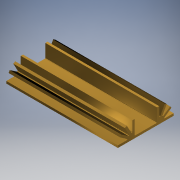
# Autodesk Inventor part: ZD3-5 Disipador
Saved by Autodesk Inventor 2018.3 (Build 223284000, 284)
## iProperties
Created: 2021-05-04
Part Number: ZD3-5 Disipador
Material: Latón, amarillo claro
Document SubType Name: Modeling
Designer: laguerre
Density: 8.47 g/cm^3
Appearance: Latón - Satinado
Author: laguerre
Autodesk Inventor part; units mm, degrees
ref_plane "YZ Plane" through (0, 0, 0) normal (1, 0, 0) x (0, 1, 0)
ref_plane "XZ Plane" through (0, 0, 0) normal (0, 1, 0) x (-1, 0, 0)
ref_plane "XY Plane" through (0, 0, 0) normal (0, 0, 1) x (1, 0, 0)
sketch "Boceto39" plane through (0, 0, 0) normal (0, 0, 1) x (1, 0, 0)
  line L0 (-25, 0) -> (25, 0)
  line L1 (10, 15) -> (10, 2.5)
  line L2 (9.5, 2) -> (-9.5, 2)
  line L3 (10, 15) -> (12, 15)
  line L4 (12, 15) -> (12, 6)
  line L5 (12.9398, 5.7622) -> (16.9826, 13.2392)
  line L6 (16.9826, 13.2392) -> (18.7419, 12.288)
  line L7 (18.7419, 12.288) -> (14.947, 5.2693)
  line L8 (15.67, 4.6194) -> (21.8509, 8.8675)
  line L9 (21.8509, 8.8675) -> (22.9837, 7.2192)
  line L10 (22.9837, 7.2192) -> (16.7168, 2.9121)
  line L11 (17, 2) -> (25, 2)
  line L12 (25, 2) -> (25, 0)
  line L13 (-10, 2.5) -> (-10, 14)
  line L14 (-10, 14) -> (-12, 14)
  line L15 (-17, 2) -> (-25, 2)
  line L16 (-25, 2) -> (-25, 0)
  arc A0 (25, 0) -> (10, 15) centre (10, 0) ccw construction
  line L17 (-12, 14) -> (-12, 6)
  line L18 (-12.9398, 5.7622) -> (-16.9826, 13.2392)
  line L19 (-16.9826, 13.2392) -> (-18.7419, 12.288)
  line L20 (-18.7419, 12.288) -> (-14.947, 5.2693)
  line L21 (-15.67, 4.6194) -> (-21.8509, 8.8675)
  line L22 (-21.8509, 8.8675) -> (-22.9837, 7.2192)
  line L23 (-22.9837, 7.2192) -> (-16.7168, 2.9121)
  arc A1 (-12.9398, 5.7622) -> (-12, 6) centre (-12.5, 6) ccw
  arc A2 (-15.67, 4.6194) -> (-14.947, 5.2693) centre (-15.3868, 5.0315) ccw
  arc A3 (-17, 2) -> (-16.7168, 2.9121) centre (-17, 2.5) ccw
  arc A4 (12, 6) -> (12.9398, 5.7622) centre (12.5, 6) ccw
  arc A5 (14.947, 5.2693) -> (15.67, 4.6194) centre (15.3868, 5.0315) ccw
  arc A6 (16.7168, 2.9121) -> (17, 2) centre (17, 2.5) ccw
  arc A7 (9.5, 2) -> (10, 2.5) centre (9.5, 2.5) ccw
  arc A8 (-10, 2.5) -> (-9.5, 2) centre (-9.5, 2.5) ccw
  point P0 (0, 0)
  point P1 (0, 0)
  dimension "d373" = 50
  dimension "d374" = 2
  dimension "d375" = 14
  dimension "d376" = 10
  dimension "d377" = 10
  dimension "d378" = 28.4
  dimension "d379" = 27.1
  dimension "d380" = 28.4
  dimension "d381" = 27.1
  dimension "d382" = 0.5
  dimension "d383" = 4
  dimension "d384" = 17
  dimension "d385" = 17
  dimension "d386" = 8.5
  dimension "d387" = 7.5
  constraints: 48 end point, 18 point on circle, 18 tangent, 10 perpendicular, 9 centre point, 8 equal length, 7 equal radius, 4 vertical, 3 parallel, 2 collinear, 2 horizontal, 1 coincident, 1 horizontal alignment, 1 midpoint
  measures "d373" distance of L0.start L0.end
  measures "d374" distance between parallel lines of L0 L2
  measures "d375" distance between parallel lines of L0 L14
  measures "d376" distance from line of point (0, 0) L13
  measures "d377" distance from line of point (0, 0) L1
  measures "d378" angle of L5 L4
  measures "d379" angle of L8 L7
  measures "d380" angle of L18 L17
  measures "d381" angle of L21 L20
  measures "d382" radius of A1
  measures "d383" distance from line of A4.centre L2
  measures "d384" horizontal distance of point (0, 0) A6.centre
  measures "d385" horizontal distance of point (0, 0) A3.centre
  measures "d386" distance of L5.start L5.end
  measures "d387" distance of L8.start L8.end
extrude "Extrusión13" add sketch "Boceto39" along normal mid plane 100
sketch "Boceto40" plane through (-9.5, 2, 50) normal (0, 1, 0) x (1, 0, 0)
  line L0 (9.5, 18) -> (9.5, 18) construction
  line L1 (9.5, 18) -> (9.5, 82) construction
  line L2 (9.5, 82) -> (9.5, 82) construction
  line L3 (9.5, 82) -> (9.5, 18) construction
  point P0 (9.5, 50)
  point P1 (9.5, 82)
  point P2 (9.5, 50)
  dimension "d390" = 0
  dimension "d391" = 64
  constraints: 8 end point, 5 coincident, 2 equal length, 2 midpoint, 1 horizontal, 1 perpendicular, 1 vertical alignment
  measures "d390" distance of L1.end L2.end
  measures "d391" distance of L2.end L0.start
hole "Agujero2" at (0, 2, 32) at (0, 2, 32) at (0, 2, -32) at (0, 2, -32) direction (0, -1, 0) diameter 3 depth 8 tip angle 118
